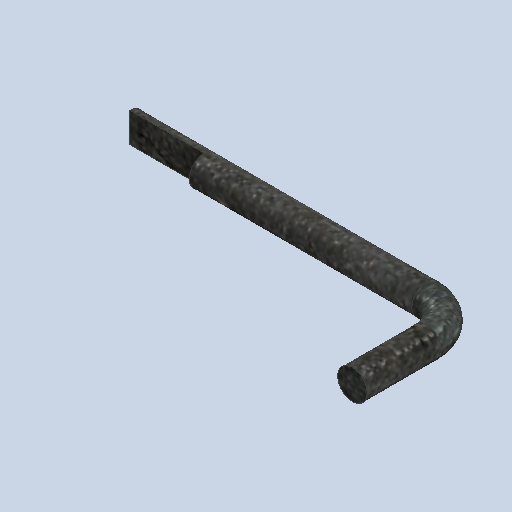
# Autodesk Inventor part: AllenKey-RS3
Saved by Autodesk Inventor 2024.3 (Build 283343000, 343)
## iProperties
Created: 2025-07-31
Part Number: AllenKey-RS3
Material: Steel
Document SubType Name: Modeling
Designer: ajclo
Density: 7.85 g/cm^3
Appearance: Plate
Mass: 41.7107 g
Surface Area: 29.1726 cm^2
Volume: 5.31346 cm^3
Author: ajclo
Autodesk Inventor part; units mm, degrees
ref_plane "YZ Plane" through (0, 0, 0) normal (1, 0, 0) x (0, 1, 0)
ref_plane "XZ Plane" through (0, 0, 0) normal (0, 1, 0) x (-1, 0, 0)
ref_plane "XY Plane" through (0, 0, 0) normal (0, 0, 1) x (1, 0, 0)
sketch "Sketch1" plane through (0, 0, 0) normal (1, 0, 0) x (0, 1, 0)
  circle A0 centre (0, 0) radius 4
  dimension "d0" = 8
  constraints: 1 centre point, 1 coincident
  measures "d0" diameter of A0
extrude "Extrusion1" add sketch "Sketch1" along normal blind 80
sketch "Sketch8" plane through (80, 0, 0) normal (1, 0, 0) x (0, 0, -1)
  line L0 (-10, -3.7509) -> (-10, 5.6543)
  circle A0 centre (0, 0) radius 4 projected
  point P0 (-10, 0.9517)
  dimension "d13" = 10
  constraints: 2 end point, 1 midpoint, 1 vertical
  measures "d13" horizontal distance of point (0, 0) point (-10, 0.952)
revolve "Revolution2" add sketch "Sketch8" angle 90 about axis through (80, -3.7509, 10) along (0, -1, 0)
sketch "Sketch9" plane through (90, 0, 10) normal (0, 0, 1) x (1, 0, 0)
  circle A0 centre (0, 0) radius 4 projected
  point P0 (-90, 0)
extrude "Extrusion6" add sketch "Sketch9" along normal blind 20
sketch "Sketch10" plane through (0, 0, 0) normal (-1, 0, 0) x (0, 0, 1)
  circle A0 centre (0, 0) radius 4 projected
  line L0 (0, -4.7151) -> (0, 4)
  point P0 (0, -4)
  constraints: 2 end point, 2 other
extrude "Extrusion7" cut sketch "Sketch10" against normal blind 20 contours A0 L0 picked at (0.5785, 1.2013)
body "Solid1"
